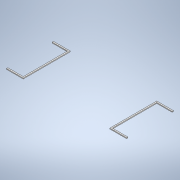
# Autodesk Inventor part: Place_of_goalKipeer
Saved by Autodesk Inventor 2020 (Build 240168000, 168)
## iProperties
Created: 2022-01-17
Part Number: Place_of_goalKipeer
Material: Типовые
Document SubType Name: Modeling
Designer: Администратор
Density: 1 g/cm^3
Appearance: По умолчанию
Author: Администратор
Autodesk Inventor part; units mm, degrees
ref_plane "YZ Plane" through (0, 0, 0) normal (1, 0, 0) x (0, 1, 0)
ref_plane "XZ Plane" through (0, 0, 0) normal (0, 1, 0) x (-1, 0, 0)
ref_plane "XY Plane" through (0, 0, 0) normal (0, 0, 1) x (1, 0, 0)
sketch "Эскиз1" plane through (0, 0, 0) normal (0, 1, 0) x (-1, 0, 0)
  line L0 (895, -350) -> (645, -350)
  line L1 (645, -350) -> (645, 350)
  line L2 (645, 350) -> (895, 350)
  line L3 (0, -490) -> (0, 490) construction
  line L4 (1463.2221, 0) -> (-1288.037, 0) construction
  line L5 (895, 330) -> (665, 330)
  line L6 (665, 330) -> (665, -330)
  line L7 (665, -330) -> (895, -330)
  line L8 (895, -350) -> (895, -330)
  line L9 (895, 330) -> (895, 350)
  line L10 (-895, -350) -> (-645, -350)
  line L11 (-645, -350) -> (-645, 350)
  line L12 (-645, 350) -> (-895, 350)
  line L13 (-895, 330) -> (-665, 330)
  line L14 (-665, 330) -> (-665, -330)
  line L15 (-665, -330) -> (-895, -330)
  line L16 (-895, -350) -> (-895, -330)
  line L17 (-895, 330) -> (-895, 350)
  line L18 (895, -350) -> (895, 350) construction
  line L19 (895, 30) -> (1070.1851, 30)
  line L20 (1070.1851, 30) -> (1070.1851, -30)
  line L21 (1070.1851, -30) -> (895, -30)
  point P0 (0, 0)
  dimension "d0" = 250
  dimension "d1" = 700
  dimension "d2" = 645
  dimension "d3" = 20
  dimension "d6" = 60
  constraints: 40 end point, 8 symmetric about line, 3 horizontal, 3 vertical, 2 perpendicular, 2 point on line, 1 collinear, 1 parallel, 4 other
  measures "d0" distance of L0.start L0.end
  measures "d1" distance of L0.end L1.end
  measures "d2" distance between parallel lines of L3 L1
  measures "d3" distance between parallel lines of L1 L6
  measures "d6" distance of L19.end L20.end
extrude "Выдавливание1" add sketch "Эскиз1" along normal blind 12
